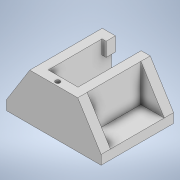
# Autodesk Inventor part: servommount1
Saved by Autodesk Inventor 2020 (Build 240168000, 168)
## iProperties
Created: 2019-08-02
Part Number: servommount1
Material: Generic
Document SubType Name: Modeling
Designer: cui_t
Density: 1 g/cm^3
Appearance: Default
Author: cui_t
Autodesk Inventor part; units mm, degrees
ref_plane "YZ Plane" through (0, 0, 0) normal (1, 0, 0) x (0, 1, 0)
ref_plane "XZ Plane" through (0, 0, 0) normal (0, 1, 0) x (-1, 0, 0)
ref_plane "XY Plane" through (0, 0, 0) normal (0, 0, 1) x (1, 0, 0)
sketch "Sketch1" plane through (0, 0, 0) normal (0, 1, 0) x (-1, 0, 0)
  point P0 (0, 0)
sketch "Sketch2" plane through (0, 0, 0) normal (0, 1, 0) x (-1, 0, 0)
  line L0 (-10.25, -15.5) -> (10.25, -15.5)
  line L1 (10.25, -15.5) -> (10.25, 15.5)
  line L2 (10.25, 15.5) -> (-10.25, 15.5)
  line L3 (-10.25, 15.5) -> (-10.25, -15.5)
  line L4 (-10.25, -15.5) -> (10.25, 15.5) construction
  line L5 (10.25, -15.5) -> (-10.25, 15.5) construction
  point P0 (0, 0)
  dimension "d0" = 20.5
  dimension "d1" = 31
  constraints: 12 end point, 2 midpoint, 2 parallel, 1 horizontal, 1 perpendicular
  measures "d0" distance of L2.end L1.end
  measures "d1" distance of L0.end L1.end
extrude "Extrusion1" add sketch "Sketch2" along normal blind 20
sketch "Sketch3" plane through (0, 20, 0) normal (0, 1, 0) x (1, 0, 0)
  line L0 (6.375, -11.5) -> (-6.375, -11.5)
  line L1 (-6.375, -11.5) -> (-6.375, 11.5)
  line L2 (-6.375, 11.5) -> (6.375, 11.5)
  line L3 (6.375, 11.5) -> (6.375, -11.5)
  line L4 (10.25, 15.5) -> (-10.25, 15.5) projected
  line L5 (10.25, -15.5) -> (10.25, 15.5) projected
  line L6 (-10.25, 15.5) -> (-10.25, -15.5) projected
  line L7 (-10.25, -15.5) -> (10.25, -15.5) projected
  point P0 (0, 0)
  dimension "d4" = 23
  dimension "d5" = 12.75
  dimension "d6" = 4
  dimension "d7" = 3.875
  dimension "d8" = 3.875
  dimension "d9" = 4
  constraints: 8 end point, 2 parallel, 1 horizontal, 1 perpendicular
  measures "d4" distance of L0.end L1.end
  measures "d5" distance of L1.end L2.end
  measures "d6" distance between parallel lines of L4 L2
  measures "d7" distance between parallel lines of L5 L3
  measures "d8" distance between parallel lines of L1 L6
  measures "d9" distance between parallel lines of L7 L0
extrude "Extrusion2" cut sketch "Sketch3" against normal blind 16 contours L0 L1 L2 L3
sketch "Sketch4" plane through (10.25, 0, -15.5) normal (0, 0, -1) x (-1, 0, 0)
  line L0 (16.625, 14) -> (3.875, 14)
  line L1 (3.875, 14) -> (3.875, 4)
  line L2 (3.875, 4) -> (16.625, 4)
  line L3 (16.625, 4) -> (16.625, 14)
  line L4 (3.875, 20) -> (16.625, 20) projected
  line L5 (0, 0) -> (20.5, 0) projected
  line L6 (0, 0) -> (0, 20) projected
  line L7 (20.5, 0) -> (20.5, 20) projected
  point P0 (10.25, 0)
  dimension "d12" = 10
  dimension "d13" = 12.75
  dimension "d14" = 4
  dimension "d15" = 3.875
  dimension "d16" = 3.875
  dimension "d17" = 6
  constraints: 8 end point, 3 parallel, 1 horizontal, 1 perpendicular
  measures "d12" distance of L2.end L0.start
  measures "d13" distance of L1.end L2.end
  measures "d14" distance between parallel lines of L5 L2
  measures "d15" distance between parallel lines of L6 L1
  measures "d16" distance between parallel lines of L7 L3
  measures "d17" distance between parallel lines of L4 L0
extrude "Extrusion3" cut sketch "Sketch4" against normal blind 4
sketch "Sketch5" plane through (0, 20, 0) normal (0, 1, 0) x (1, 0, 0)
  circle A0 centre (0, -13.8) radius 0.975
  line L0 (6.375, -11.5) -> (-6.375, -11.5) projected
  line L1 (10.25, -15.5) -> (10.25, 15.5) projected
  line L2 (-10.25, 15.5) -> (-10.25, -15.5) projected
  circle A1 centre (0, 13.8) radius 0.975
  line L3 (-6.375, 11.5) -> (6.375, 11.5) projected
  point P0 (0, 0)
  dimension "d20" = 1.95
  dimension "d21" = 2.3
  dimension "d22" = 10.25
  dimension "d23" = 10.25
  dimension "d24" = 1.95
  dimension "d25" = 2.3
  dimension "d26" = 10.25
  dimension "d27" = 10.25
  constraints: 2 centre point
  measures "d20" diameter of A0
  measures "d21" distance from line of L0 A0.centre
  measures "d22" distance from line of L1 A0.centre
  measures "d23" distance from line of L2 A0.centre
  measures "d24" diameter of A1
  measures "d25" distance from line of L3 A1.centre
  measures "d26" distance from line of L1 A1.centre
  measures "d27" distance from line of L2 A1.centre
extrude "Extrusion4" cut sketch "Sketch5" against normal blind 8
sketch "Sketch6" plane through (-10.25, 0, -15.5) normal (-1, 0, 0) x (0, 0, 1)
  line L0 (0, 4) -> (27, 4) projected
  line L1 (0, 0) -> (31, 0) projected
  line L2 (0, 4) -> (31, 4)
  line L3 (31, 4) -> (31, 0)
  line L4 (31, 0) -> (0, 0)
  line L5 (0, 0) -> (0, 4)
  point P0 (15.5, 0)
  constraints: 8 end point, 2 parallel, 1 horizontal, 1 perpendicular
extrude "Extrusion5" add sketch "Sketch6" along normal blind 10
sketch "Sketch8" plane through (10.25, 0, 15.5) normal (1, 0, 0) x (0, 0, -1)
  line L0 (31, 4) -> (4, 4) projected
  line L1 (0, 0) -> (31, 0) projected
  line L2 (31, 4) -> (0, 4)
  line L3 (0, 4) -> (0, 0)
  line L4 (0, 0) -> (31, 0)
  line L5 (31, 0) -> (31, 4)
  point P0 (15.5, 0)
  point P1 (4, 4)
  constraints: 8 end point, 2 parallel, 1 horizontal, 1 perpendicular
extrude "Extrusion6" add sketch "Sketch8" along normal blind 10
sketch "Sketch9" plane through (10.25, 20, -15.5) normal (0, 0, -1) x (-1, 0, 0)
  line L0 (20.5, -16) -> (20.5, 0) projected
  line L1 (20.5, 0) -> (20.5, -16)
  line L2 (30.5, -20) -> (30.5, -16) projected
  line L3 (20.5, -16) -> (30.5, -16)
  line L4 (30.5, -16) -> (20.5, 0)
  line L5 (0, -16) -> (0, 0) projected
  line L6 (0, 0) -> (0, -16)
  line L7 (0, -16) -> (-10, -16) projected
  line L8 (0, -16) -> (-10, -16)
  line L9 (-10, -16) -> (0, 0)
  point P0 (10.25, -20)
  constraints: 12 end point, 2 collinear, 1 perpendicular, 1 vertical
extrude "Extrusion7" add sketch "Sketch9" against normal blind 4
sketch "Sketch10" plane through (-10.25, 20, 15.5) normal (0, 0, 1) x (1, 0, 0)
  line L0 (0, 0) -> (0, -16)
  line L1 (0, -16) -> (-10, -16) projected
  line L2 (0, -16) -> (-10, -16)
  line L3 (-10, -16) -> (0, 0) projected
  line L4 (-10, -16) -> (0, 0)
  line L5 (20.5, -16) -> (20.5, 0) projected
  line L6 (20.5, 0) -> (20.5, -16)
  line L7 (20.5, -16) -> (30.5, -16) projected
  line L8 (20.5, -16) -> (30.5, -16)
  line L9 (30.5, -16) -> (20.5, 0)
  point P0 (10.25, -20)
  constraints: 12 end point, 2 perpendicular, 2 vertical, 1 collinear
extrude "Extrusion8" add sketch "Sketch10" against normal blind 4
sketch "Sketch11" plane through (0, 20, 0) normal (0, 1, 0) x (1, 0, 0)
  line L0 (6.375, 15.5) -> (6.375, -11.5) projected
  line L1 (-6.375, 11.5) -> (6.375, 11.5) projected
  line L2 (6.375, 15.5) -> (-4.625, 15.5)
  line L3 (-4.625, 15.5) -> (-4.625, 11.5)
  line L4 (-4.625, 11.5) -> (6.375, 11.5)
  line L5 (6.375, 11.5) -> (6.375, 15.5)
  point P0 (0, 0)
  dimension "d38" = 11
  constraints: 8 end point, 2 parallel, 1 horizontal, 1 perpendicular, 1 point on line
  measures "d38" distance of L4.end L3.end
extrude "Extrusion9" cut sketch "Sketch11" against normal blind 6
body "Solid1"
